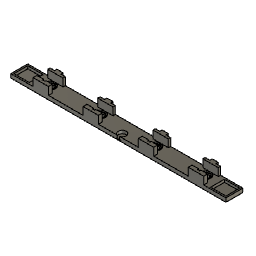
LEDHoldingMechanism (Autodesk Fusion 360 design; units mm, degrees)
Autodesk Fusion 360 part; units mm, degrees
sketch "Skizze10" plane through (0, 0, 0) normal (0, 0, 1) x (1, 0, 0)
  line L0 (140, 13) -> (-140, 13)
  line L1 (-140, 13) -> (-140, -13)
  line L2 (-140, -13) -> (140, -13)
  line L3 (140, -13) -> (140, 13)
  line L4 (140, 13) -> (-140, -13) construction
  line L5 (-140, 13) -> (140, -13) construction
  dimension "d78" = 280
  dimension "d79" = 26
  constraint horizontal L0
  constraint perpendicular L0 L1
  constraint parallel L0 L2
  constraint parallel L1 L3
  constraint coincident L4 origin
  constraint coincident L5 origin
  measures "d78" distance of L1.end L2.end
  measures "d79" distance of L0.end L1.end
extrude "Extrusion12" add sketch "Skizze10" along normal blind 5
sketch "Skizze11" plane through (0, 0, 5) normal (0, 0, 1) x (-1, 0, 0)
  line L0 (-140, 13) -> (-140, -13)
  line L1 (-140, -13) -> (140, -13)
  line L2 (140, -13) -> (140, 13)
  line L3 (140, 13) -> (-140, 13)
  circle A0 centre (0, 4) radius 5.25
  dimension "d86" = 10.5
  measures "d86" diameter of A0
sketch "Skizze12" plane through (0, 0, 0) normal (0, 0, -1) x (1, 0, 0)
  line L0 (140, -13) -> (140, 13)
  line L1 (140, 13) -> (-140, 13)
  line L2 (-140, 13) -> (-140, -13)
  line L3 (-140, -13) -> (140, -13)
  line L4 (71, -1.75) -> (1, -1.75)
  line L5 (1, -1.75) -> (1, -4.25)
  line L6 (1, -4.25) -> (71, -4.25)
  line L7 (71, -4.25) -> (71, -1.75)
  line L8 (71, -1.75) -> (1, -4.25) construction
  line L9 (1, -1.75) -> (71, -4.25) construction
  line L10 (72.9933, -1.75) -> (104.9933, -1.75)
  line L11 (104.9933, -1.75) -> (104.9933, -4.25)
  line L12 (104.9933, -4.25) -> (72.9933, -4.25)
  line L13 (72.9933, -4.25) -> (72.9933, -1.75)
  line L14 (0, 13) -> (0, -13)
  line L15 (-71, -1.75) -> (-1, -4.25) construction
  line L16 (-71, -1.75) -> (-1, -1.75)
  line L17 (-71, -4.25) -> (-71, -1.75)
  line L18 (-1, -1.75) -> (-1, -4.25)
  line L19 (-1, -1.75) -> (-71, -4.25) construction
  line L20 (-1, -4.25) -> (-71, -4.25)
  line L21 (-104.9933, -1.75) -> (-104.9933, -4.25)
  line L22 (-72.9933, -4.25) -> (-72.9933, -1.75)
  line L23 (-104.9933, -4.25) -> (-72.9933, -4.25)
  line L24 (-72.9933, -1.75) -> (-104.9933, -1.75)
  point P0 (36, -3)
  point P1 (-105, -3)
  point P2 (-36, -3)
  dimension "d87" = 70
  dimension "d88" = 2.5
  dimension "d89" = 32
  dimension "d90" = 2.5
  constraint horizontal L4
  constraint perpendicular L4 L5
  constraint parallel L4 L6
  constraint parallel L5 L7
  constraint coincident L8 P0
  constraint coincident L9 P0
  constraint horizontal L10
  constraint vertical L11
  constraint horizontal L12
  constraint vertical L13
  constraint midpoint L1 L14.start
  constraint midpoint L3 L14.end
  constraint symmetric L4.start L14 L15.start
  constraint symmetric L4.end L14 L16.end
  constraint symmetric L5.end L14 L15.end
  constraint symmetric L6.end L14 L17.start
  constraint symmetric P0 L14 P2
  constraint symmetric L10.start L14 L22.end
  constraint symmetric L10.end L14 L21.start
  constraint symmetric L11.end L14 L21.end
  constraint symmetric L12.end L14 L22.start
  measures "d87" distance of L5.end L6.end
  measures "d88" distance of L4.end L5.end
  measures "d89" distance of L10.start L10.end
  measures "d90" distance of L10.start L12.end
extrude "Extrusion13" cut sketch "Skizze11" against normal up to surface (4 mm away) contours A0
extrude "Extrusion14" cut sketch "Skizze12" against normal blind 2 contours L4 L5 L6 L7 | L10 L11 L12 L13 | L16 L17 L18 L20 | L21 L22 L23 L24
sketch "Skizze13" plane through (0, 0, 5) normal (0, 0, 1) x (-1, 0, 0)
  circle A0 centre (0, 4) radius 5.25
  line L0 (-140, 13) -> (-140, -13)
  line L1 (-140, -13) -> (140, -13)
  line L2 (140, -13) -> (140, 13)
  line L3 (140, 13) -> (-140, 13)
  line L4 (33.25, -5.75) -> (38.75, -5.75)
  line L5 (38.75, -5.75) -> (38.75, -0.25)
  line L6 (38.75, -0.25) -> (33.25, -0.25)
  line L7 (33.25, -0.25) -> (33.25, -5.75)
  line L8 (33.25, -5.75) -> (38.75, -0.25) construction
  line L9 (38.75, -5.75) -> (33.25, -0.25) construction
  line L10 (-33.25, -5.75) -> (-38.75, -5.75)
  line L11 (-38.75, -5.75) -> (-38.75, -0.25)
  line L12 (-38.75, -0.25) -> (-33.25, -0.25)
  line L13 (-33.25, -0.25) -> (-33.25, -5.75)
  line L14 (-33.25, -5.75) -> (-38.75, -0.25) construction
  line L15 (-38.75, -5.75) -> (-33.25, -0.25) construction
  line L16 (-103.75, -5.75) -> (-98.25, -5.75)
  line L17 (-98.25, -5.75) -> (-98.25, -0.25)
  line L18 (-98.25, -0.25) -> (-103.75, -0.25)
  line L19 (-103.75, -0.25) -> (-103.75, -5.75)
  line L20 (-103.75, -5.75) -> (-98.25, -0.25) construction
  line L21 (-98.25, -5.75) -> (-103.75, -0.25) construction
  line L22 (98.25, -5.75) -> (103.75, -5.75)
  line L23 (103.75, -5.75) -> (103.75, -0.25)
  line L24 (103.75, -0.25) -> (98.25, -0.25)
  line L25 (98.25, -0.25) -> (98.25, -5.75)
  line L26 (98.25, -5.75) -> (103.75, -0.25) construction
  line L27 (103.75, -5.75) -> (98.25, -0.25) construction
  line L28 (96.5, -7.5) -> (105.5, -7.5)
  line L29 (105.5, -7.5) -> (105.5, 1.5)
  line L30 (105.5, 1.5) -> (96.5, 1.5)
  line L31 (96.5, 1.5) -> (96.5, -7.5)
  line L32 (96.5, -7.5) -> (105.5, 1.5) construction
  line L33 (105.5, -7.5) -> (96.5, 1.5) construction
  line L34 (31.5, -7.5) -> (40.5, -7.5)
  line L35 (40.5, -7.5) -> (40.5, 1.5)
  line L36 (40.5, 1.5) -> (31.5, 1.5)
  line L37 (31.5, 1.5) -> (31.5, -7.5)
  line L38 (31.5, -7.5) -> (40.5, 1.5) construction
  line L39 (40.5, -7.5) -> (31.5, 1.5) construction
  line L40 (-40.5, -7.5) -> (-31.5, -7.5)
  line L41 (-31.5, -7.5) -> (-31.5, 1.5)
  line L42 (-31.5, 1.5) -> (-40.5, 1.5)
  line L43 (-40.5, 1.5) -> (-40.5, -7.5)
  line L44 (-40.5, -7.5) -> (-31.5, 1.5) construction
  line L45 (-31.5, -7.5) -> (-40.5, 1.5) construction
  line L46 (-105.5, -7.5) -> (-96.5, -7.5)
  line L47 (-96.5, -7.5) -> (-96.5, 1.5)
  line L48 (-96.5, 1.5) -> (-105.5, 1.5)
  line L49 (-105.5, 1.5) -> (-105.5, -7.5)
  line L50 (-105.5, -7.5) -> (-96.5, 1.5) construction
  line L51 (-96.5, -7.5) -> (-105.5, 1.5) construction
  line L52 (103.75, -5.75) -> (98.25, -5.75)
  line L53 (98.25, -5.75) -> (98.25, -7.5)
  line L54 (98.25, -7.5) -> (103.75, -7.5)
  line L55 (103.75, -7.5) -> (103.75, -5.75)
  line L56 (103.75, -0.25) -> (98.25, -0.25)
  line L57 (98.25, -0.25) -> (98.25, 1.5)
  line L58 (98.25, 1.5) -> (103.75, 1.5)
  line L59 (103.75, 1.5) -> (103.75, -0.25)
  line L60 (38.75, -0.25) -> (33.25, -0.25)
  line L61 (33.25, -0.25) -> (33.25, 1.5)
  line L62 (33.25, 1.5) -> (38.75, 1.5)
  line L63 (38.75, 1.5) -> (38.75, -0.25)
  line L64 (38.75, -5.75) -> (33.25, -5.75)
  line L65 (33.25, -5.75) -> (33.25, -7.5)
  line L66 (33.25, -7.5) -> (38.75, -7.5)
  line L67 (38.75, -7.5) -> (38.75, -5.75)
  line L68 (-33.25, -0.25) -> (-38.75, -0.25)
  line L69 (-38.75, -0.25) -> (-38.75, 1.5)
  line L70 (-38.75, 1.5) -> (-33.25, 1.5)
  line L71 (-33.25, 1.5) -> (-33.25, -0.25)
  line L72 (-33.25, -5.75) -> (-38.75, -5.75)
  line L73 (-38.75, -5.75) -> (-38.75, -7.5)
  line L74 (-38.75, -7.5) -> (-33.25, -7.5)
  line L75 (-33.25, -7.5) -> (-33.25, -5.75)
  line L76 (-98.25, -0.25) -> (-103.75, -0.25)
  line L77 (-103.75, -0.25) -> (-103.75, 1.5)
  line L78 (-103.75, 1.5) -> (-98.25, 1.5)
  line L79 (-98.25, 1.5) -> (-98.25, -0.25)
  line L80 (-98.25, -5.75) -> (-103.75, -5.75)
  line L81 (-103.75, -5.75) -> (-103.75, -7.5)
  line L82 (-103.75, -7.5) -> (-98.25, -7.5)
  line L83 (-98.25, -7.5) -> (-98.25, -5.75)
  point P0 (36, -3)
  point P1 (-36, -3)
  point P2 (-101, -3)
  point P3 (101, -3)
  point P4 (101, -3)
  point P5 (36, -3)
  point P6 (-36, -3)
  point P7 (-101, -3)
  dimension "d95" = 5.5
  dimension "d96" = 5.5
  dimension "d97" = 5.5
  dimension "d98" = 5.5
  dimension "d99" = 5.5
  dimension "d100" = 5.5
  dimension "d101" = 5.5
  dimension "d102" = 5.5
  dimension "d165" = 9
  dimension "d166" = 9
  dimension "d167" = 9
  dimension "d168" = 9
  dimension "d169" = 9
  dimension "d170" = 9
  dimension "d171" = 9
  dimension "d172" = 9
  dimension "d175" = 5.5
  dimension "d176" = 5.5
  dimension "d177" = 5.5
  dimension "d178" = 5.5
  dimension "d179" = 5.5
  dimension "d180" = 5.5
  dimension "d181" = 5.5
  dimension "d182" = 5.5
  constraint horizontal L4
  constraint perpendicular L4 L5
  constraint parallel L4 L6
  constraint parallel L5 L7
  constraint coincident L8 P5
  constraint coincident L9 P5
  constraint horizontal L10
  constraint perpendicular L10 L11
  constraint parallel L10 L12
  constraint parallel L11 L13
  constraint coincident L14 P6
  constraint coincident L15 P6
  constraint horizontal L16
  constraint perpendicular L16 L17
  constraint parallel L16 L18
  constraint parallel L17 L19
  constraint coincident L20 P7
  constraint coincident L21 P7
  constraint horizontal L22
  constraint perpendicular L22 L23
  constraint parallel L22 L24
  constraint parallel L23 L25
  constraint coincident L26 P4
  constraint coincident L27 P4
  constraint horizontal L28
  constraint perpendicular L28 L29
  constraint parallel L28 L30
  constraint parallel L29 L31
  constraint coincident L32 P4
  constraint coincident L33 P4
  constraint coincident P4 P3
  constraint horizontal L34
  constraint perpendicular L34 L35
  constraint parallel L34 L36
  constraint parallel L35 L37
  constraint coincident L38 P5
  constraint coincident L39 P5
  constraint coincident P5 P0
  constraint horizontal L40
  constraint perpendicular L40 L41
  constraint parallel L40 L42
  constraint parallel L41 L43
  constraint coincident L44 P6
  constraint coincident L45 P6
  constraint coincident P6 P1
  constraint horizontal L46
  constraint perpendicular L46 L47
  constraint parallel L46 L48
  constraint parallel L47 L49
  constraint coincident L50 P7
  constraint coincident L51 P7
  constraint coincident P7 P2
  constraint horizontal L52
  constraint vertical L53
  constraint horizontal L54
  constraint vertical L55
  constraint horizontal L56
  constraint vertical L57
  constraint horizontal L58
  constraint vertical L59
  constraint horizontal L60
  constraint vertical L61
  constraint horizontal L62
  constraint vertical L63
  constraint horizontal L64
  constraint vertical L65
  constraint horizontal L66
  constraint vertical L67
  constraint horizontal L68
  constraint vertical L69
  constraint horizontal L70
  constraint vertical L71
  constraint horizontal L72
  constraint vertical L73
  constraint horizontal L74
  constraint vertical L75
  constraint horizontal L76
  constraint vertical L77
  constraint horizontal L78
  constraint vertical L79
  constraint horizontal L80
  constraint vertical L81
  constraint horizontal L82
  constraint vertical L83
  measures "d95" distance of L5.end L6.end
  measures "d96" distance of L4.end L5.end
  measures "d97" distance of L11.end L12.end
  measures "d98" distance of L10.end L11.end
  measures "d99" distance of L17.end L18.end
  measures "d100" distance of L16.end L17.end
  measures "d101" distance of L23.end L24.end
  measures "d102" distance of L22.end L23.end
  measures "d165" distance of L29.end L30.end
  measures "d166" distance of L28.end L29.end
  measures "d167" distance of L35.end L36.end
  measures "d168" distance of L34.end L35.end
  measures "d169" distance of L41.end L42.end
  measures "d170" distance of L40.end L41.end
  measures "d171" distance of L47.end L48.end
  measures "d172" distance of L46.end L47.end
  measures "d175" distance of L22.end L22.start
  measures "d176" distance of L23.end L24.end
  measures "d177" distance of L5.end L6.end
  measures "d178" distance of L4.end L4.start
  measures "d179" distance of L12.end L11.end
  measures "d180" distance of L10.start L10.end
  measures "d181" distance of L17.end L18.end
  measures "d182" distance of L16.end L16.start
extrude "Extrusion25" cut sketch "Skizze13" against normal blind 2.5 contours L7 L34 L36 L37 L61 L65 | L5 L34 L35 L36 L63 L67 | L13 L40 L41 L42 L71 L75 | L11 L40 L42 L43 L69 L73 | L19 L46 L48 L49 L77 L81 | L17 L46 L47 L48 L79 L83 | L25 L28 L30 L31 L53 L57 | L23 L28 L29 L30 L55 L59
extrude "Extrusion24" cut sketch "Skizze13" against normal blind 1.5 contours L7 L34 L36 L37 L61 L65 | L4 L34 L64 L65 L66 L67 | L5 L34 L35 L36 L63 L67 | L6 L36 L60 L61 L62 L63 | L10 L40 L72 L73 L74 L75 | L13 L40 L41 L42 L71 L75 | L11 L40 L42 L43 L69 L73 | L12 L42 L68 L69 L70 L71 | L19 L46 L48 L49 L77 L81 | L16 L46 L80 L81 L82 L83 | L17 L46 L47 L48 L79 L83 | L18 L48 L76 L77 L78 L79 | L25 L28 L30 L31 L53 L57 | L22 L28 L52 L53 L54 L55 | L23 L28 L29 L30 L55 L59 | L24 L30 L56 L57 L58 L59
extrude "Extrusion15" cut sketch "Skizze13" against normal blind 5 contours L4 L5 L6 L7 L60 L64 | L10 L11 L12 L13 L68 L72 | L16 L17 L18 L19 L76 L80 | L22 L23 L24 L25 L52 L56
sketch "Skizze14" plane through (0, 0, 5) normal (0, 0, 1) x (-1, 0, 0)
  circle A0 centre (0, 4) radius 5.25
  line L0 (-140, 13) -> (-140, -13)
  line L1 (-140, -13) -> (140, -13)
  line L2 (140, -13) -> (140, 13)
  line L3 (140, 13) -> (-140, 13)
  circle A1 centre (101, -3) radius 7
  circle A2 centre (36, -3) radius 7
  circle A3 centre (-36, -3) radius 7
  circle A4 centre (-101, -3) radius 7
  line L4 (-31.5, -7.5) -> (-40.5, -7.5)
  line L5 (-40.5, -7.5) -> (-40.5, 1.5)
  line L6 (-40.5, 1.5) -> (-31.5, 1.5)
  line L7 (-31.5, 1.5) -> (-31.5, -7.5)
  line L8 (40.5, -7.5) -> (31.5, -7.5)
  line L9 (31.5, -7.5) -> (31.5, 1.5)
  line L10 (31.5, 1.5) -> (40.5, 1.5)
  line L11 (40.5, 1.5) -> (40.5, -7.5)
  line L12 (-96.5, -7.5) -> (-105.5, -7.5)
  line L13 (-105.5, -7.5) -> (-105.5, 1.5)
  line L14 (-105.5, 1.5) -> (-96.5, 1.5)
  line L15 (-96.5, 1.5) -> (-96.5, -7.5)
  line L16 (105.5, -7.5) -> (96.5, -7.5)
  line L17 (96.5, -7.5) -> (96.5, 1.5)
  line L18 (96.5, 1.5) -> (105.5, 1.5)
  line L19 (105.5, 1.5) -> (105.5, -7.5)
  dimension "d105" = 14
  dimension "d106" = 14
  dimension "d107" = 14
  dimension "d108" = 14
  measures "d105" diameter of A1
  measures "d106" diameter of A2
  measures "d107" diameter of A3
  measures "d108" diameter of A4
extrude "Extrusion16" cut sketch "Skizze14" against normal blind 1.5 contours A1 | A2 | A3 | A4 | L4 L5 L6 L7 | L8 L9 L10 L11 | L12 L13 L14 L15 | L16 L17 L18 L19
sketch "Skizze21" plane through (0, 0, 3.5) normal (0, 0, 1) x (-1, 0, 0)
  circle A0 centre (-101, -3) radius 7
  line L0 (-98.25, -0.25) -> (-98.25, 1.5)
  line L1 (-98.25, 1.5) -> (-96.5, 1.5)
  line L2 (-96.5, 1.5) -> (-96.5, -7.5)
  line L3 (-96.5, -7.5) -> (-98.25, -7.5)
  line L4 (-98.25, -7.5) -> (-98.25, -5.75)
  line L5 (-98.25, -5.75) -> (-103.75, -5.75)
  line L6 (-103.75, -5.75) -> (-103.75, -7.5)
  line L7 (-103.75, -7.5) -> (-105.5, -7.5)
  line L8 (-105.5, -7.5) -> (-105.5, 1.5)
  line L9 (-105.5, 1.5) -> (-103.75, 1.5)
  line L10 (-103.75, 1.5) -> (-103.75, -0.25)
  line L11 (-103.75, -0.25) -> (-98.25, -0.25)
  line L12 (-98.25, -5.75) -> (-103.75, -5.75)
  line L13 (-103.75, -5.75) -> (-103.75, -7.5)
  line L14 (-103.75, -7.5) -> (-98.25, -7.5)
  line L15 (-98.25, -7.5) -> (-98.25, -5.75)
  line L16 (-98.25, -0.25) -> (-103.75, -0.25)
  line L17 (-103.75, -0.25) -> (-103.75, 1.5)
  line L18 (-103.75, 1.5) -> (-98.25, 1.5)
  line L19 (-98.25, 1.5) -> (-98.25, -0.25)
  constraint horizontal L12
  constraint vertical L13
  constraint horizontal L14
  constraint vertical L15
  constraint coincident L6.end L7.start
  constraint coincident L4.end L5.start
  constraint horizontal L16
  constraint vertical L17
  constraint horizontal L18
  constraint vertical L19
  constraint coincident L9.end L10.start
  constraint coincident L0.start L11.end
sketch "Skizze22" plane through (0, 0, 3.5) normal (0, 0, 1) x (-1, 0, 0)
  circle A0 centre (-36, -3) radius 7
  line L0 (-33.25, -0.25) -> (-33.25, 1.5)
  line L1 (-33.25, 1.5) -> (-31.5, 1.5)
  line L2 (-31.5, 1.5) -> (-31.5, -7.5)
  line L3 (-31.5, -7.5) -> (-33.25, -7.5)
  line L4 (-33.25, -7.5) -> (-33.25, -5.75)
  line L5 (-33.25, -5.75) -> (-38.75, -5.75)
  line L6 (-38.75, -5.75) -> (-38.75, -7.5)
  line L7 (-38.75, -7.5) -> (-40.5, -7.5)
  line L8 (-40.5, -7.5) -> (-40.5, 1.5)
  line L9 (-40.5, 1.5) -> (-38.75, 1.5)
  line L10 (-38.75, 1.5) -> (-38.75, -0.25)
  line L11 (-38.75, -0.25) -> (-33.25, -0.25)
  line L12 (-33.25, -0.25) -> (-38.75, -0.25)
  line L13 (-38.75, -0.25) -> (-38.75, 1.5)
  line L14 (-38.75, 1.5) -> (-33.25, 1.5)
  line L15 (-33.25, 1.5) -> (-33.25, -0.25)
  line L16 (-33.25, -5.75) -> (-38.75, -5.75)
  line L17 (-38.75, -5.75) -> (-38.75, -7.5)
  line L18 (-38.75, -7.5) -> (-33.25, -7.5)
  line L19 (-33.25, -7.5) -> (-33.25, -5.75)
  constraint horizontal L12
  constraint vertical L13
  constraint horizontal L14
  constraint vertical L15
  constraint coincident L9.end L10.start
  constraint coincident L0.start L11.end
  constraint horizontal L16
  constraint vertical L17
  constraint horizontal L18
  constraint vertical L19
  constraint coincident L6.end L7.start
  constraint coincident L4.end L5.start
sketch "Skizze23" plane through (0, 0, 3.5) normal (0, 0, 1) x (-1, 0, 0)
  circle A0 centre (36, -3) radius 7
  line L0 (33.25, 1.5) -> (33.25, -0.25)
  line L1 (33.25, -0.25) -> (38.75, -0.25)
  line L2 (38.75, -0.25) -> (38.75, 1.5)
  line L3 (38.75, 1.5) -> (40.5, 1.5)
  line L4 (40.5, 1.5) -> (40.5, -7.5)
  line L5 (40.5, -7.5) -> (38.75, -7.5)
  line L6 (38.75, -7.5) -> (38.75, -5.75)
  line L7 (38.75, -5.75) -> (33.25, -5.75)
  line L8 (33.25, -5.75) -> (33.25, -7.5)
  line L9 (33.25, -7.5) -> (31.5, -7.5)
  line L10 (31.5, -7.5) -> (31.5, 1.5)
  line L11 (31.5, 1.5) -> (33.25, 1.5)
  line L12 (38.75, -0.25) -> (33.25, -0.25)
  line L13 (33.25, -0.25) -> (33.25, 1.5)
  line L14 (33.25, 1.5) -> (38.75, 1.5)
  line L15 (38.75, 1.5) -> (38.75, -0.25)
  line L16 (38.75, -5.75) -> (33.25, -5.75)
  line L17 (33.25, -5.75) -> (33.25, -7.5)
  line L18 (33.25, -7.5) -> (38.75, -7.5)
  line L19 (38.75, -7.5) -> (38.75, -5.75)
  constraint horizontal L12
  constraint vertical L13
  constraint horizontal L14
  constraint vertical L15
  constraint coincident L0.start L11.end
  constraint coincident L1.end L2.start
  constraint horizontal L16
  constraint vertical L17
  constraint horizontal L18
  constraint vertical L19
  constraint coincident L8.end L9.start
  constraint coincident L6.end L7.start
sketch "Skizze24" plane through (0, 0, 3.5) normal (0, 0, 1) x (-1, 0, 0)
  circle A0 centre (101, -3) radius 7
  line L0 (103.75, -0.25) -> (103.75, 1.5)
  line L1 (103.75, 1.5) -> (105.5, 1.5)
  line L2 (105.5, 1.5) -> (105.5, -7.5)
  line L3 (105.5, -7.5) -> (103.75, -7.5)
  line L4 (103.75, -7.5) -> (103.75, -5.75)
  line L5 (103.75, -5.75) -> (98.25, -5.75)
  line L6 (98.25, -5.75) -> (98.25, -7.5)
  line L7 (98.25, -7.5) -> (96.5, -7.5)
  line L8 (96.5, -7.5) -> (96.5, 1.5)
  line L9 (96.5, 1.5) -> (98.25, 1.5)
  line L10 (98.25, 1.5) -> (98.25, -0.25)
  line L11 (98.25, -0.25) -> (103.75, -0.25)
  line L12 (103.75, -0.25) -> (98.25, -0.25)
  line L13 (98.25, -0.25) -> (98.25, 1.5)
  line L14 (98.25, 1.5) -> (103.75, 1.5)
  line L15 (103.75, 1.5) -> (103.75, -0.25)
  line L16 (103.75, -5.75) -> (98.25, -5.75)
  line L17 (98.25, -5.75) -> (98.25, -7.5)
  line L18 (98.25, -7.5) -> (103.75, -7.5)
  line L19 (103.75, -7.5) -> (103.75, -5.75)
  constraint horizontal L12
  constraint vertical L13
  constraint horizontal L14
  constraint vertical L15
  constraint coincident L9.end L10.start
  constraint coincident L0.start L11.end
  constraint horizontal L16
  constraint vertical L17
  constraint horizontal L18
  constraint vertical L19
  constraint coincident L6.end L7.start
  constraint coincident L4.end L5.start
extrude "Extrusion26" add sketch "Skizze21" sketch "Skizze22" sketch "Skizze23" sketch "Skizze24" along normal blind 1 contours L0 L10 L11 L16 L17 L18 L19 | L4 L5 L6 L12 L13 L14 L15 of sketch 2 contours L0 L10 L11 L12 L13 L14 L15 | L4 L5 L6 L16 L17 L18 L19 of sketch 3 contours L0 L1 L2 L12 L13 L14 L15 | L6 L7 L8 L16 L17 L18 L19 of sketch 4 contours L0 L10 L11 L12 L13 L14 L15 | L4 L5 L6 L16 L17 L18 L19
sketch "Skizze25" plane through (0, 0, 5) normal (0, 0, 1) x (-1, 0, 0)
  circle A0 centre (-36, -3) radius 7
  circle A1 centre (36, -3) radius 7
  circle A2 centre (-101, -3) radius 7
  circle A3 centre (101, -3) radius 7
  line L0 (-140, 13) -> (-140, -13)
  line L1 (-140, -13) -> (140, -13)
  line L2 (140, -13) -> (140, 13)
  line L3 (140, 13) -> (-140, 13)
  circle A4 centre (0, 4) radius 5.25
  line L4 (91, -13) -> (111, -13)
  line L5 (111, -13) -> (111, -10)
  line L6 (111, -10) -> (91, -10)
  line L7 (91, -10) -> (91, -13)
  line L8 (91, -13) -> (111, -10) construction
  line L9 (111, -13) -> (91, -10) construction
  line L10 (91, 4) -> (111, 4)
  line L11 (111, 4) -> (111, 7)
  line L12 (111, 7) -> (91, 7)
  line L13 (91, 7) -> (91, 4)
  line L14 (91, 4) -> (111, 7) construction
  line L15 (111, 4) -> (91, 7) construction
  line L16 (26, -13) -> (46, -13)
  line L17 (46, -13) -> (46, -10)
  line L18 (46, -10) -> (26, -10)
  line L19 (26, -10) -> (26, -13)
  line L20 (26, -13) -> (46, -10) construction
  line L21 (46, -13) -> (26, -10) construction
  line L22 (26, 4) -> (46, 4)
  line L23 (46, 4) -> (46, 7)
  line L24 (46, 7) -> (26, 7)
  line L25 (26, 7) -> (26, 4)
  line L26 (26, 4) -> (46, 7) construction
  line L27 (46, 4) -> (26, 7) construction
  line L28 (-46, -13) -> (-26, -13)
  line L29 (-26, -13) -> (-26, -10)
  line L30 (-26, -10) -> (-46, -10)
  line L31 (-46, -10) -> (-46, -13)
  line L32 (-46, -13) -> (-26, -10) construction
  line L33 (-26, -13) -> (-46, -10) construction
  line L34 (-46, 4) -> (-26, 4)
  line L35 (-26, 4) -> (-26, 7)
  line L36 (-26, 7) -> (-46, 7)
  line L37 (-46, 7) -> (-46, 4)
  line L38 (-46, 4) -> (-26, 7) construction
  line L39 (-26, 4) -> (-46, 7) construction
  line L40 (-111, -13) -> (-91, -13)
  line L41 (-91, -13) -> (-91, -10)
  line L42 (-91, -10) -> (-111, -10)
  line L43 (-111, -10) -> (-111, -13)
  line L44 (-111, -13) -> (-91, -10) construction
  line L45 (-91, -13) -> (-111, -10) construction
  line L46 (-111, 4) -> (-91, 4)
  line L47 (-91, 4) -> (-91, 7)
  line L48 (-91, 7) -> (-111, 7)
  line L49 (-111, 7) -> (-111, 4)
  line L50 (-111, 4) -> (-91, 7) construction
  line L51 (-91, 4) -> (-111, 7) construction
  point P0 (101, -11.5)
  point P1 (101, 5.5)
  point P2 (36, -11.5)
  point P3 (36, 5.5)
  point P4 (-36, -11.5)
  point P5 (-36, 5.5)
  point P6 (-101, -11.5)
  point P7 (-101, 5.5)
  dimension "d187" = 20
  dimension "d188" = 20
  dimension "d189" = 20
  dimension "d190" = 3
  dimension "d191" = 20
  dimension "d192" = 3
  dimension "d193" = 20
  dimension "d194" = 3
  dimension "d195" = 20
  dimension "d196" = 20
  dimension "d197" = 3
  dimension "d198" = 20
  dimension "d199" = 3
  constraint horizontal L4
  constraint perpendicular L4 L5
  constraint parallel L4 L6
  constraint parallel L5 L7
  constraint coincident L8 P0
  constraint coincident L9 P0
  constraint horizontal L10
  constraint perpendicular L10 L11
  constraint parallel L10 L12
  constraint parallel L11 L13
  constraint coincident L14 P1
  constraint coincident L15 P1
  constraint horizontal L16
  constraint perpendicular L16 L17
  constraint parallel L16 L18
  constraint parallel L17 L19
  constraint coincident L20 P2
  constraint coincident L21 P2
  constraint horizontal L22
  constraint perpendicular L22 L23
  constraint parallel L22 L24
  constraint parallel L23 L25
  constraint coincident L26 P3
  constraint coincident L27 P3
  constraint horizontal L28
  constraint perpendicular L28 L29
  constraint parallel L28 L30
  constraint parallel L29 L31
  constraint coincident L32 P4
  constraint coincident L33 P4
  constraint horizontal L34
  constraint perpendicular L34 L35
  constraint parallel L34 L36
  constraint parallel L35 L37
  constraint coincident L38 P5
  constraint coincident L39 P5
  constraint horizontal L40
  constraint perpendicular L40 L41
  constraint parallel L40 L42
  constraint parallel L41 L43
  constraint coincident L44 P6
  constraint coincident L45 P6
  constraint horizontal L46
  constraint perpendicular L46 L47
  constraint parallel L46 L48
  constraint parallel L47 L49
  constraint coincident L50 P7
  constraint coincident L51 P7
  measures "d187" distance of L5.end L6.end
  measures "d188" distance of L11.end L12.end
  measures "d189" distance of L17.end L18.end
  measures "d190" distance of L16.end L17.end
  measures "d191" distance of L23.end L24.end
  measures "d192" distance of L22.end L23.end
  measures "d193" distance of L29.end L30.end
  measures "d194" distance of L28.end L29.end
  measures "d195" distance of L35.end L36.end
  measures "d196" distance of L41.end L42.end
  measures "d197" distance of L40.end L41.end
  measures "d198" distance of L47.end L48.end
  measures "d199" distance of L46.end L47.end
extrude "Extrusion27" add sketch "Skizze25" along normal blind 10 contours L22 L23 L24 L25 | L10 L11 L12 L13 | L46 L47 L48 L49 | L1 L28 L29 L30 L31 | L34 L35 L36 L37 | L1 L16 L17 L18 L19 | L1 L40 L41 L42 L43 | L1 L4 L5 L6 L7
move_face "Flächen versetzen11" offset 0.1 16 faces at (-104.1644, 1.75, 0.6667) (-81.4122, 1.75, 1.3333) (-60.25, 1.75, 0.6667) (-22.5, 1.75, 1.3333) (22.5, 1.75, 1.3333) (60.25, 1.75, 0.6667) (81.4122, 1.75, 0.6667) (104.1644, 1.75, 0.6667) (104.5788, 4.25, 0.6667) (89.8311, 4.25, 0.6667) (49.5, 4.25, 1.3333) (11.75, 4.25, 0.6667) (-11.75, 4.25, 0.6667) (-49.5, 4.25, 1.3333) (-89.8311, 4.25, 0.6667) (-104.5788, 4.25, 0.6667)
move_face "Flächen versetzen12" offset 2 4 faces at (-104.3333, -7, 8.3333) (-39.3333, -7, 8.3333) (32.6667, -7, 8.3333) (97.6667, -7, 8.3333)
sketch "Skizze26" plane through (0, -4, 0) normal (0, 1, 0) x (-1, 0, 0)
  line L0 (-111, 5) -> (-101, 5)
  line L1 (-101, 5) -> (-91, 5)
  line L2 (-91, 5) -> (-91, 15)
  line L3 (-91, 15) -> (-111, 15)
  line L4 (-111, 15) -> (-111, 5)
  line L5 (-99.5, 8) -> (-102.5, 8)
  line L6 (-102.5, 8) -> (-102.5, 15)
  line L7 (-102.5, 15) -> (-99.5, 15)
  line L8 (-99.5, 15) -> (-99.5, 8)
  line L9 (-37.5, 8) -> (-34.5, 8)
  line L10 (-34.5, 8) -> (-34.5, 15)
  line L11 (-34.5, 15) -> (-37.5, 15)
  line L12 (-37.5, 15) -> (-37.5, 8)
  line L13 (34.5, 8) -> (37.5, 8)
  line L14 (37.5, 8) -> (37.5, 15)
  line L15 (37.5, 15) -> (34.5, 15)
  line L16 (34.5, 15) -> (34.5, 8)
  line L17 (99.5, 8) -> (102.5, 8)
  line L18 (102.5, 8) -> (102.5, 15)
  line L19 (102.5, 15) -> (99.5, 15)
  line L20 (99.5, 15) -> (99.5, 8)
  dimension "d204" = 3
  constraint horizontal L5
  constraint vertical L6
  constraint horizontal L7
  constraint vertical L8
  constraint horizontal L9
  constraint vertical L10
  constraint horizontal L11
  constraint vertical L12
  constraint horizontal L13
  constraint vertical L14
  constraint horizontal L15
  constraint vertical L16
  constraint horizontal L17
  constraint vertical L18
  constraint horizontal L19
  constraint vertical L20
  measures "d204" distance of L5.start L5.end
extrude "Extrusion28" cut sketch "Skizze26" against normal blind 1.5 contours L3 L5 L6 L7 L8 | L9 L10 L11 L12 | L13 L14 L15 L16 | L17 L18 L19 L20
sketch "Skizze27" plane through (0, 13, 0) normal (0, 1, 0) x (-1, 0, 0)
  line L0 (-140, 0) -> (140, 0)
  line L1 (140, 0) -> (140, 5)
  line L2 (140, 5) -> (111, 5)
  line L3 (111, 5) -> (111, 15)
  line L4 (111, 15) -> (91, 15)
  line L5 (91, 15) -> (91, 5)
  line L6 (91, 5) -> (46, 5)
  line L7 (46, 5) -> (46, 15)
  line L8 (46, 15) -> (26, 15)
  line L9 (26, 15) -> (26, 5)
  line L10 (26, 5) -> (-26, 5)
  line L11 (-26, 5) -> (-26, 15)
  line L12 (-26, 15) -> (-46, 15)
  line L13 (-46, 15) -> (-46, 5)
  line L14 (-46, 5) -> (-91, 5)
  line L15 (-91, 5) -> (-91, 15)
  line L16 (-91, 15) -> (-111, 15)
  line L17 (-111, 15) -> (-111, 5)
  line L18 (-111, 5) -> (-140, 5)
  line L19 (-140, 5) -> (-140, 0)
  line L20 (40, 14) -> (32, 14)
  line L21 (32, 14) -> (32, 0)
  line L22 (32, 0) -> (40, 0)
  line L23 (40, 0) -> (40, 14)
  line L24 (40, 14) -> (32, 0) construction
  line L25 (32, 14) -> (40, 0) construction
  line L26 (105, 14) -> (97, 14)
  line L27 (97, 14) -> (97, 0)
  line L28 (97, 0) -> (105, 0)
  line L29 (105, 0) -> (105, 14)
  line L30 (105, 14) -> (97, 0) construction
  line L31 (97, 14) -> (105, 0) construction
  line L32 (-32, 14) -> (-40, 14)
  line L33 (-40, 14) -> (-40, 0)
  line L34 (-40, 0) -> (-32, 0)
  line L35 (-32, 0) -> (-32, 14)
  line L36 (-32, 14) -> (-40, 0) construction
  line L37 (-40, 14) -> (-32, 0) construction
  line L38 (-97, 14) -> (-105, 14)
  line L39 (-105, 14) -> (-105, 0)
  line L40 (-105, 0) -> (-97, 0)
  line L41 (-97, 0) -> (-97, 14)
  line L42 (-97, 14) -> (-105, 0) construction
  line L43 (-105, 14) -> (-97, 0) construction
  point P0 (36, 7)
  point P1 (101, 7)
  point P2 (-36, 7)
  point P3 (-101, 7)
  constraint horizontal L20
  constraint perpendicular L20 L21
  constraint parallel L20 L22
  constraint parallel L21 L23
  constraint coincident L24 P0
  constraint coincident L25 P0
  constraint horizontal L26
  constraint perpendicular L26 L27
  constraint parallel L26 L28
  constraint parallel L27 L29
  constraint coincident L30 P1
  constraint coincident L31 P1
  constraint horizontal L32
  constraint perpendicular L32 L33
  constraint parallel L32 L34
  constraint parallel L33 L35
  constraint coincident L36 P2
  constraint coincident L37 P2
  constraint horizontal L38
  constraint perpendicular L38 L39
  constraint parallel L38 L40
  constraint parallel L39 L41
  constraint coincident L42 P3
  constraint coincident L43 P3
extrude "Extrusion29" add sketch "Skizze27" along normal blind 3 contours L0 L38 L39 L40 L41 | L0 L32 L33 L34 L35 | L0 L20 L21 L22 L23 | L0 L26 L27 L28 L29
move_face "Flächen versetzen13" offset -0.25 4 faces at (1, 3.3833, 1.3333) (-1, 3.3833, 1.3333) (-71, 2.6167, 1.3333) (71, 2.6167, 1.3333)
move_face "Flächen versetzen14" offset 1 4 faces at (-37.3333, 14, 14) (34.6667, 14, 14) (99.6667, 14, 14) (-102.3333, 14, 14)
move_face "Flächen versetzen15" offset -4 1 faces at (-46.6667, -13, 1.6667)
sketch "Skizze28" plane through (0, 0, 5) normal (0, 0, 1) x (-1, 0, 0)
  line L0 (-111, 4) -> (-111, 9)
  line L1 (-111, 9) -> (-140, 9)
  line L2 (-140, 9) -> (-140, -13)
  line L3 (-140, -13) -> (-111, -13)
  line L4 (-111, -13) -> (-111, -10)
  line L5 (-111, -10) -> (-101, -10)
  arc A0 (-101, 4) -> (-101, -10) centre (-101, -3) ccw
  line L6 (-101, 4) -> (-111, 4)
  line L7 (-138, -11) -> (-118, -11)
  line L8 (-118, -11) -> (-118, 7)
  line L9 (-118, 7) -> (-138, 7)
  line L10 (-138, 7) -> (-138, -11)
  line L11 (138, -11) -> (118, -11)
  line L12 (118, -11) -> (118, 7)
  line L13 (118, 7) -> (138, 7)
  line L14 (138, 7) -> (138, -11)
  dimension "d212" = 20
  dimension "d213" = 18
  dimension "d214" = 20
  dimension "d215" = 18
  constraint horizontal L7
  constraint vertical L8
  constraint horizontal L9
  constraint vertical L10
  constraint horizontal L11
  constraint vertical L12
  constraint horizontal L13
  constraint vertical L14
  measures "d212" distance of L7.start L7.end
  measures "d213" distance of L7.start L9.end
  measures "d214" distance of L11.start L11.end
  measures "d215" distance of L11.start L13.end
extrude "Extrusion30" cut sketch "Skizze28" against normal up to surface (3.5 mm away) contours L7 L8 L9 L10 | L11 L12 L13 L14
